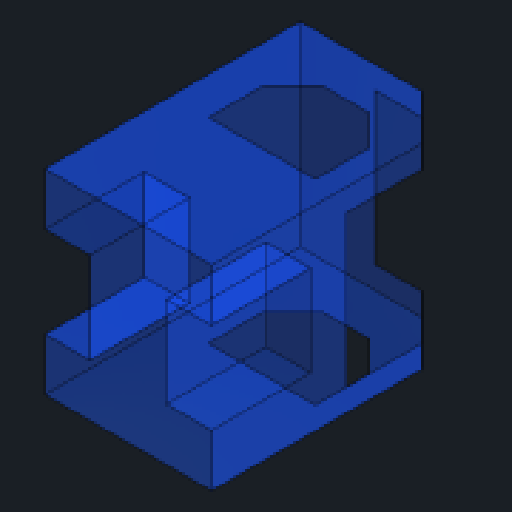
# Autodesk Inventor part: Croqui Célula
Saved by Autodesk Inventor 2026 (Build 300175000, 175)
## iProperties
Created: 2025-06-19
Part Number: Croqui Célula
Material: Genérico
Document SubType Name: Modeling
Designer: WANDREW
Mass: 12777.8 g
Surface Area: 170597 cm^2
Volume: 12777.8 cm^3
Density: 1 g/cm^3
Appearance: Transparente - Azul
Author: WANDREW
Autodesk Inventor part; units mm, degrees
ref_plane "YZ Plane" through (0, 0, 0) normal (1, 0, 0) x (0, 1, 0)
ref_plane "XZ Plane" through (0, 0, 0) normal (0, 1, 0) x (-1, 0, 0)
ref_plane "XY Plane" through (0, 0, 0) normal (0, 0, 1) x (1, 0, 0)
sketch "Esboço1" plane through (0, 0, 0) normal (0, 0, 1) x (1, 0, 0)
  line L0 (555, 651.5) -> (-555, 651.5)
  line L1 (-555, 651.5) -> (-555, -651.5)
  line L2 (-555, -651.5) -> (555, -651.5)
  line L3 (555, -651.5) -> (555, 651.5)
  point P0 (0, 0)
  point P1 (555, 0)
  point P2 (0, 651.5)
  dimension "d11" = 1110
  dimension "d12" = 1303
  constraints: 8 end point, 2 midpoint, 2 parallel, 1 horizontal, 1 horizontal alignment, 1 perpendicular, 1 vertical alignment
  measures "d11" distance between parallel lines of L3 L1
  measures "d12" distance between parallel lines of L2 L0
extrude "Extrusão1" add sketch "Esboço1" against normal blind 1700
sketch "Esboço3" plane through (-555, -651.5, 0) normal (0, -1, 0) x (1, 0, 0)
  line L0 (960, -1400) -> (250, -1400)
  line L1 (250, -1400) -> (250, -840)
  line L2 (250, -840) -> (960, -840)
  line L3 (960, -840) -> (960, -1400)
  line L4 (1110, 0) -> (1110, -1700) construction
  line L5 (0, 0) -> (0, -1700) construction
  line L6 (1110, -1700) -> (0, -1700) projected
  line L7 (1110, 0) -> (0, 0) construction
  point P0 (555, 0)
  dimension "d2" = 150
  dimension "d3" = 250
  dimension "d4" = 300
  dimension "d10" = 560
  dimension "d17" = 840
  constraints: 8 end point, 2 parallel, 1 horizontal, 1 perpendicular
  measures "d2" distance between parallel lines of L4 L3
  measures "d3" distance between parallel lines of L5 L1
  measures "d4" distance between parallel lines of L6 L0
  measures "d10" distance of L2.end L0.start
  measures "d17" distance between parallel lines of L7 L2
extrude "Extrusão2" cut sketch "Esboço3" against normal through all
chamfer "Chanfro2" distance 300 angle 45 1 edges at (555, 0, -1700)
chamfer "Chanfro1" distance 200 angle 45 2 edges at (-305, 0, -1400) (405, 0, -1400)
sketch "Esboço4" plane through (555, -651.5, 0) normal (1, 0, 0) x (0, 0, -1)
  line L0 (0, 1303) -> (0, 0) projected
  line L1 (660, 952.5) -> (0, 952.5)
  line L2 (0, 952.5) -> (0, 350.5)
  line L3 (0, 350.5) -> (660, 350.5)
  line L4 (660, 350.5) -> (660, 952.5)
  line L5 (0, 1303) -> (1400, 1303) projected
  line L6 (0, 0) -> (1400, 0) projected
  point P0 (0, 651.5)
  point P1 (0, 952.5)
  dimension "d19" = 350.5
  dimension "d20" = 350.5
  dimension "d21" = 660
  dimension "d22" = 602
  constraints: 8 end point, 2 parallel, 1 horizontal, 1 perpendicular, 1 point on line
  measures "d19" distance between parallel lines of L5 L1
  measures "d20" distance between parallel lines of L6 L3
  measures "d21" distance of L2.end L3.end
  measures "d22" distance of L3.end L1.start
extrude "Extrusão3" cut sketch "Esboço4" against normal blind 300
sketch "Esboço6" plane through (-555, -651.5, 0) normal (-1, 0, 0) x (0, 0, 1)
  line L0 (-660, 349) -> (0, 349)
  line L1 (0, 349) -> (0, 954)
  line L2 (0, 954) -> (-660, 954)
  line L3 (-660, 954) -> (-660, 349)
  line L4 (0, 1303) -> (0, 0) projected
  line L5 (0, 952.5) -> (-660, 952.5) projected
  point P0 (0, 651.5)
  point P1 (0, 651.5)
  dimension "d30" = 660
  dimension "d31" = 660
  dimension "d32" = 605
  constraints: 8 end point, 2 midpoint, 2 parallel, 1 horizontal, 1 perpendicular
  measures "d30" distance of L1.end L2.end
  measures "d31" distance from line of L4 L5.end
  measures "d32" distance between parallel lines of L0 L2
extrude "Extrusão5" cut sketch "Esboço6" against normal blind 300 contours L3 L5 L1 L0
shell "Casca1" thickness 1.5 removed faces 7 at (85, 534.6667, 0) at (168.3333, -217.1667, -840) at (-305, 217.1667, -960) at (-238.3333, -217.1667, -1266.6667) at (-1.6667, -217.1667, -1400) at (405, -217.1667, -1080) at (271.6667, -217.1667, -1333.3333)
sketch "Esboço5" plane through (0, 0, -1700) normal (0, 0, -1) x (-1, 0, 0)
  line L0 (55, 501.5) -> (-555, 501.5)
  line L1 (-555, 501.5) -> (-555, -501.5)
  line L2 (-555, -501.5) -> (55, -501.5)
  line L3 (55, -501.5) -> (55, 501.5)
  line L4 (-255, 651.5) -> (-555, 651.5) construction
  line L5 (-255, -651.5) -> (555, -651.5) construction
  line L6 (-555, 651.5) -> (-555, -651.5) construction
  line L7 (555, -651.5) -> (555, 651.5) construction
  line L8 (555, 651.5) -> (-555, 651.5)
  line L9 (-555, 651.5) -> (-555, -651.5)
  line L10 (-555, -651.5) -> (555, -651.5)
  line L11 (555, -651.5) -> (555, 651.5)
  point P0 (0, 0)
  dimension "d25" = 150
  dimension "d26" = 150
  dimension "d27" = 500
  constraints: 16 end point, 4 parallel, 2 horizontal, 2 perpendicular, 1 point on line
  measures "d25" distance between parallel lines of L0 L4
  measures "d26" distance between parallel lines of L2 L5
  measures "d27" distance between parallel lines of L7 L3
extrude "Extrusão4" cut sketch "Esboço5" against normal blind 800 contours L3 L2 L1 L0
sketch "Esboço7" plane through (255, -651.5, 0) normal (1, 0, 0) x (0, 0, -1)
  line L0 (661.5, 349) -> (0, 349) construction
  line L1 (440, 952.5) -> (435, 952.5)
  line L2 (435, 952.5) -> (435, 349)
  line L3 (435, 349) -> (440, 349)
  line L4 (440, 349) -> (440, 952.5)
  line L5 (0, 952.5) -> (660, 952.5) construction
  line L6 (0, 350.5) -> (0, 952.5) construction
  line L7 (660, 350.5) -> (0, 350.5) construction
  line L8 (660, 952.5) -> (660, 350.5) construction
  line L9 (0, 952.5) -> (660, 952.5) projected
  line L10 (215, 952.5) -> (210, 952.5)
  line L11 (210, 952.5) -> (210, 350.5)
  line L12 (210, 350.5) -> (215, 350.5)
  line L13 (215, 350.5) -> (215, 952.5)
  point P0 (0, 651.5)
  point P1 (437.5, 952.5)
  dimension "d35" = 5
  dimension "d36" = 220
  dimension "d37" = 220
  constraints: 16 end point, 5 parallel, 4 point on line, 2 horizontal, 2 perpendicular, 1 midpoint
  measures "d35" distance between parallel lines of L2 L4
  measures "d36" distance between parallel lines of L2 L13
  measures "d37" distance between parallel lines of L8 L4
equation "\"d20\" = d19"
equation "\"d26\" = d25"
equation "\"d36\" = d37"
